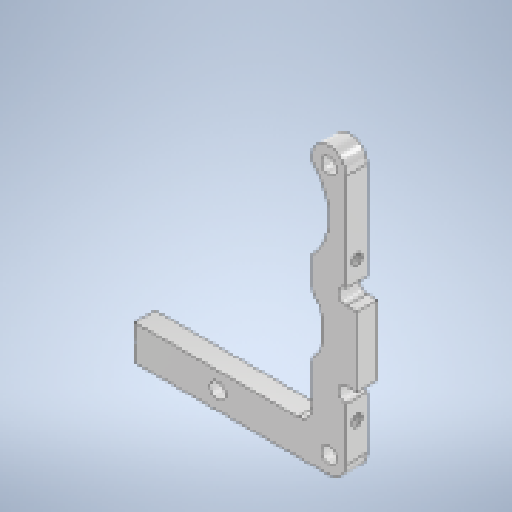
# Autodesk Inventor part: mata3
Saved by Autodesk Inventor 2025.1 (Build 291241000, 241)
## iProperties
Created: 2024-09-02
Part Number: mata3
Material: アルミニウム 2014-T4
Document SubType Name: Modeling
Designer: right
Density: 2.8 g/cm^3
Appearance: サテン
Mass: 2.43356 g
Surface Area: 11.6912 cm^2
Volume: 0.869129 cm^3
Author: right
Autodesk Inventor part; units mm, degrees
ref_plane "YZ Plane" through (0, 0, 0) normal (1, 0, 0) x (0, 1, 0)
ref_plane "XZ Plane" through (0, 0, 0) normal (0, 1, 0) x (-1, 0, 0)
ref_plane "XY Plane" through (0, 0, 0) normal (0, 0, 1) x (1, 0, 0)
sketch "スケッチ1" plane through (0, 0, 0) normal (0, 0, 1) x (1, 0, 0)
  circle A0 centre (20, -42) radius 1 projected
  circle A1 centre (4, -42) radius 1 projected
  circle A2 centre (20, -6) radius 1 projected
  circle A3 centre (20, -42) radius 1.1
  line L0 (22.5, -78.2) -> (22.5, -32.2) projected
  circle A4 centre (20, -42) radius 2.5
  circle A5 centre (20, -6) radius 2.5
  circle A6 centre (20, -6) radius 1.1
  circle A7 centre (4, -42) radius 1.1
  circle A8 centre (4, -42) radius 2.5
  line L1 (-8, -45.7) -> (-8, -64.7) projected
  line L2 (-8, -44.5) -> (-8, -39.5)
  line L3 (17.5, -42) -> (17.5, -6)
  line L4 (20, -39.5) -> (-8, -39.5)
  line L5 (20, -44.5) -> (4, -44.5)
  line L6 (4, -44.5) -> (-8, -44.5)
  line L7 (24, -24.4) -> (24, -30) projected
  line L8 (24, -32.2) -> (22.5, -32.2) projected
  line L9 (24, -22.2) -> (22.5, -22.2) projected
  line L10 (24, -32.2) -> (22.5, -32.2)
  line L11 (22.5, -32.2) -> (22.5, -22.2)
  line L12 (22.5, -22.2) -> (24, -22.2)
  line L13 (24, -22.2) -> (24, -32.2)
  line L14 (22.5, -22.2) -> (22.5, -6)
  line L15 (2, -43.5) -> (2, -4.5) projected
  arc A9 (2, -43.5) -> (2.5, -44) centre (2.5, -43.5) ccw projected
  line L16 (21.5, -44) -> (2.5, -44) projected
  arc A10 (21.5, -44) -> (22, -43.5) centre (21.5, -43.5) ccw projected
  line L17 (22, -4.5) -> (22, -43.5) projected
  arc A11 (22, -4.5) -> (21.5, -4) centre (21.5, -4.5) ccw projected
  line L18 (2.5, -4) -> (21.5, -4) projected
  arc A12 (2.5, -4) -> (2, -4.5) centre (2.5, -4.5) ccw projected
  line L19 (18.4286, -23.8214) -> (18.4286, -30.1786) projected
  line L20 (18.4286, -30.1786) -> (14.5714, -30.1786) projected
  line L21 (14.5714, -30.1786) -> (14.5714, -23.8214) projected
  line L22 (14.5714, -23.8214) -> (18.4286, -23.8214) projected
  circle A13 centre (12, -31.4) radius 1.1519 projected
  line L23 (5.5714, -23.8214) -> (9.4286, -23.8214) projected
  line L24 (9.4286, -23.8214) -> (9.4286, -30.1786) projected
  line L25 (9.4286, -30.1786) -> (5.5714, -30.1786) projected
  line L26 (5.5714, -30.1786) -> (5.5714, -23.8214) projected
  circle A14 centre (20, -6) radius 1.8131 projected
  circle A15 centre (4, -6) radius 1.8131 projected
  circle A16 centre (20, -42) radius 1.8131 projected
  circle A17 centre (4, -42) radius 1.8131 projected
  arc A18 (18.25, -12.4893) -> (5.75, -12.5) centre (12, -12.5) ccw projected
  arc A19 (18.5, -12.25) -> (18.2502, -12.4893) centre (18.5, -12.5) ccw projected
  line L27 (18.5, -12.25) -> (20.25, -12.25) projected
  arc A20 (20.25, -12.75) -> (20.25, -12.25) centre (20.25, -12.5) ccw projected
  line L28 (20.25, -12.75) -> (18.5, -12.75) projected
  arc A21 (18.25, -12.5) -> (18.5, -12.75) centre (18.5, -12.5) ccw projected
  arc A22 (17.7742, -14.8918) -> (18.25, -12.5) centre (12, -12.5) ccw projected
  arc A23 (18.1009, -14.7565) -> (17.7742, -14.8918) centre (18.0052, -14.9874) ccw projected
  line L29 (18.1009, -14.7565) -> (19.7177, -15.4262) projected
  arc A24 (19.5263, -15.8881) -> (19.7177, -15.4262) centre (19.622, -15.6571) ccw projected
  line L30 (19.5263, -15.8881) -> (17.9095, -15.2184) projected
  arc A25 (17.7742, -14.8918) -> (17.9095, -15.2184) centre (18.0052, -14.9874) ccw projected
  arc A26 (16.4194, -16.9194) -> (17.7742, -14.8918) centre (12, -12.5) ccw projected
  arc A27 (16.773, -16.9194) -> (16.4194, -16.9194) centre (16.5962, -17.0962) ccw projected
  line L31 (16.773, -16.9194) -> (18.0104, -18.1569) projected
  arc A28 (17.6569, -18.5104) -> (18.0104, -18.1569) centre (17.8336, -18.3336) ccw projected
  line L32 (17.6569, -18.5104) -> (16.4194, -17.273) projected
  arc A29 (16.4194, -16.9194) -> (16.4194, -17.273) centre (16.5962, -17.0962) ccw projected
  arc A30 (14.3918, -18.2742) -> (16.4194, -16.9194) centre (12, -12.5) ccw projected
  arc A31 (14.7184, -18.4095) -> (14.3918, -18.2742) centre (14.4874, -18.5052) ccw projected
  line L33 (14.7184, -18.4095) -> (15.3881, -20.0263) projected
  arc A32 (14.9262, -20.2177) -> (15.3881, -20.0263) centre (15.1571, -20.122) ccw projected
  line L34 (14.9262, -20.2177) -> (14.2565, -18.6009) projected
  arc A33 (14.3918, -18.2742) -> (14.2565, -18.6009) centre (14.4874, -18.5052) ccw projected
  arc A34 (12, -18.75) -> (14.3918, -18.2742) centre (12, -12.5) ccw projected
  arc A35 (12.25, -19) -> (12, -18.75) centre (12, -19) ccw projected
  line L35 (12.25, -19) -> (12.25, -20.75) projected
  arc A36 (11.75, -20.75) -> (12.25, -20.75) centre (12, -20.75) ccw projected
  line L36 (11.75, -20.75) -> (11.75, -19) projected
  arc A37 (12, -18.75) -> (11.75, -19) centre (12, -19) ccw projected
  arc A38 (9.6082, -18.2742) -> (12, -18.75) centre (12, -12.5) ccw projected
  arc A39 (9.7435, -18.6009) -> (9.6082, -18.2742) centre (9.5126, -18.5052) ccw projected
  line L37 (9.7435, -18.6009) -> (9.0738, -20.2177) projected
  arc A40 (8.6119, -20.0263) -> (9.0738, -20.2177) centre (8.8429, -20.122) ccw projected
  line L38 (8.6119, -20.0263) -> (9.2816, -18.4095) projected
  arc A41 (9.6082, -18.2742) -> (9.2816, -18.4095) centre (9.5126, -18.5052) ccw projected
  arc A42 (7.5806, -16.9194) -> (9.6082, -18.2742) centre (12, -12.5) ccw projected
  arc A43 (7.5806, -17.273) -> (7.5806, -16.9194) centre (7.4038, -17.0962) ccw projected
  line L39 (7.5806, -17.273) -> (6.3431, -18.5104) projected
  arc A44 (5.9896, -18.1569) -> (6.3431, -18.5104) centre (6.1664, -18.3336) ccw projected
  line L40 (5.9896, -18.1569) -> (7.227, -16.9194) projected
  arc A45 (7.5806, -16.9194) -> (7.227, -16.9194) centre (7.4038, -17.0962) ccw projected
  arc A46 (6.2258, -14.8918) -> (7.5806, -16.9194) centre (12, -12.5) ccw projected
  arc A47 (6.0905, -15.2184) -> (6.2258, -14.8918) centre (5.9948, -14.9874) ccw projected
  line L41 (6.0905, -15.2184) -> (4.4737, -15.8881) projected
  arc A48 (4.2823, -15.4262) -> (4.4737, -15.8881) centre (4.378, -15.6571) ccw projected
  line L42 (4.2823, -15.4262) -> (5.8991, -14.7565) projected
  arc A49 (6.2258, -14.8918) -> (5.8991, -14.7565) centre (5.9948, -14.9874) ccw projected
  arc A50 (5.75, -12.5) -> (6.2258, -14.8918) centre (12, -12.5) ccw projected
  arc A51 (5.5, -12.75) -> (5.75, -12.5) centre (5.5, -12.5) ccw projected
  line L43 (5.5, -12.75) -> (3.75, -12.75) projected
  arc A52 (3.75, -12.25) -> (3.75, -12.75) centre (3.75, -12.5) ccw projected
  line L44 (3.75, -12.25) -> (5.5, -12.25) projected
  arc A53 (5.75, -12.5) -> (5.5, -12.25) centre (5.5, -12.5) ccw projected
  line L45 (18.9286, -30.6786) -> (18.9286, -23.3214)
  line L46 (18.9286, -23.3214) -> (14.0714, -23.3214)
  line L47 (14.0714, -23.3214) -> (14.0714, -30.6786)
  line L48 (14.0714, -30.6786) -> (18.9286, -30.6786)
  circle A54 centre (22.5, -21.1) radius 1.1
  circle A55 centre (22.5, -33.3) radius 1.1
  circle A56 centre (-9, -42) radius 1.1
  circle A57 centre (12, -12.5) radius 6.25
  circle A58 centre (12, -12.5) radius 8
  point P0 (0, 0)
  point P1 (-8, -42)
  point P2 (-8, -41.5417)
  point P3 (-8, -42.4583)
  point P4 (22.5, -42)
  point P5 (22.5, -34.4)
  point P6 (22.5, -20)
  point P7 (17.5, -9.5314)
  point P8 (18.25, -12.5)
  point P9 (17.5, -15.4686)
  point P10 (17.5, -17.6464)
  point P11 (17.5, -18.3536)
  point P12 (17.5, -23.3214)
  point P13 (17.5, -30.6786)
  point P14 (17.5, -39.5)
  point P15 (17.5, -6.6905)
  point P16 (17.5, -18.3095)
  dimension "d0" = 2.2
  dimension "d1" = 2.2
  dimension "d2" = 2.2
  dimension "d3" = 0.5
  dimension "d4" = 2.2
  dimension "d5" = 2.2
  dimension "d6" = 2.2
  dimension "d7" = 1
  constraints: 28 end point, 11 centre point, 10 tangent, 7 coincident, 6 point on circle, 3 equal radius, 3 point on line, 2 parallel, 1 horizontal, 1 horizontal alignment, 1 midpoint, 1 perpendicular, 1 vertical, 1 vertical alignment, 5 other
  measures "d0" diameter of A3
  measures "d1" diameter of A6
  measures "d2" diameter of A7
  measures "d3" distance between parallel lines of L19 L45
  measures "d4" diameter of A54
  measures "d5" diameter of A55
  measures "d6" diameter of A56
  measures "d7" distance from line of L2 A56.centre
extrude "押し出し1" add sketch "スケッチ1" along normal blind 3 contours A4 L17 A55 L0 | A4 L17 | A4 L16 L17 | A4 L4 L3 L48 L45 L46 L32 A28 L31 A58 L30 A24 L29 L28 A20 L27 A5 L17 A54 A55 | L11 L9 L13 L7 L8 | A55 L17 A54 L11 | A4 L16 | A4 L3 L4 | L5 A8 L16 A4 | L16 A8 L4 L3 A4 | A54 L17 A5 L14 | L6 L2 A56 L4 L15 A8 A9 | A8 L16 | L16 A8 L15 | A8 L15 L4 | A5 L17 | A9 A8 | L15 A8 | L17 A5 A58 L18 | L18 A5 | A58 L3 A5 | L27 A20 L28 A58 | L3 A58 L31 A28 L32 | L29 A24 L30 A58 | A14 | A16 | A17
fillet "フィレット1" radius 2 4 edges at (17.5, -30.6786, 1.5) (18.9286, -30.6786, 1.5) (17.5, -23.3214, 1.5) (18.9286, -23.3214, 1.5)
sketch "スケッチ2" plane through (22.5, -42, 0) normal (1, 0, 0) x (0, 0, -1)
  circle A0 centre (-1.5, 24.8) radius 1.1 projected
  circle A1 centre (-1.5, 4.8) radius 1.1 projected
  point P0 (0, 42)
  constraints: 2 coincident
hole "穴1" at (22.5, -17.2, 1.5) at (22.5, -37.2, 1.5) direction (-1, 0, 0) diameter 1.567 depth 6.3 tip angle 118 thread size "M2x0.4" class "6H" standard "ISO Metric profile"
sketch "スケッチ3" plane through (-8, -44.5, 0) normal (-1, 0, 0) x (0, 0, 1)
  line L0 (0, 2.5) -> (3, 2.5) projected
  point P0 (0, 44.5)
  point P1 (1.5, 2.5)
  constraints: 1 midpoint
hole "穴2" at (-8, -42, 1.5) direction (1, 0, 0) diameter 1.567 depth 6.3 tip angle 118 thread size "M2x0.4" class "6H" standard "ISO Metric profile"
fillet "フィレット2" radius 2 1 edges at (17.5, -39.5, 1.5)
